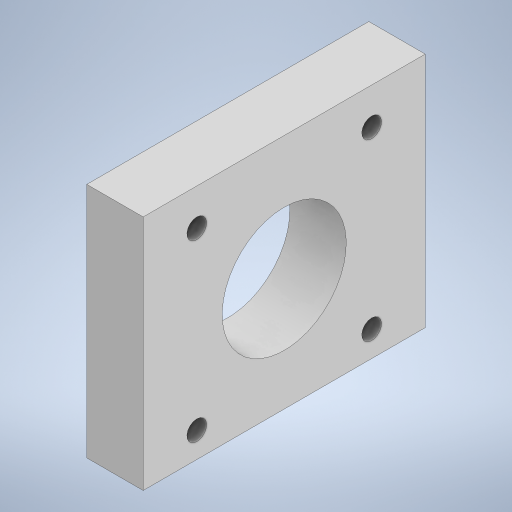
# Autodesk Inventor part: staffa motore
Saved by Autodesk Inventor 2024 (Build 280153000, 153)
## iProperties
Created: 2024-03-01
Part Number: staffa motore
Material: Generico
Document SubType Name: Modeling
Designer: Giorgio
Density: 1 g/cm^3
Appearance: Default
Author: Giorgio
Autodesk Inventor part; units mm, degrees
ref_plane "YZ Plane" through (0, 0, 0) normal (1, 0, 0) x (0, 1, 0)
ref_plane "XZ Plane" through (0, 0, 0) normal (0, 1, 0) x (-1, 0, 0)
ref_plane "XY Plane" through (0, 0, 0) normal (0, 0, 1) x (1, 0, 0)
sketch "Schizzo1" plane through (0, 0, 0) normal (1, 0, 0) x (0, 1, 0)
  circle A0 centre (57.5242, -67.0257) radius 11
  line L0 (37.5242, -92.0257) -> (79.5242, -92.0257)
  line L1 (79.5242, -92.0257) -> (79.5242, -42.0257)
  line L2 (79.5242, -42.0257) -> (37.5242, -42.0257)
  line L3 (37.5242, -42.0257) -> (37.5242, -92.0257)
  circle A1 centre (42.0242, -82.5257) radius 1.75
  circle A2 centre (42.0242, -51.5257) radius 1.75
  circle A3 centre (73.0242, -51.5257) radius 1.75
  circle A4 centre (73.0242, -82.5257) radius 1.75
  point P0 (0, 0)
  point P1 (79.5242, -67.0257)
  dimension "d0" = 22
  dimension "d1" = 42
  dimension "d2" = 50
  dimension "d4" = 31
  dimension "d5" = 31
  dimension "d6" = 15.5
  dimension "d7" = 31
  dimension "d8" = 31
  dimension "d9" = 0
  dimension "d10" = 15.5
  dimension "d11" = 0
  dimension "d12" = 3.5
  dimension "d13" = 3.5
  dimension "d14" = 3.5
  dimension "d15" = 3.5
  dimension "d16" = 22
  dimension "d17" = 25
  constraints: 8 end point, 5 centre point, 2 parallel, 1 horizontal, 1 midpoint, 1 perpendicular
  measures "d0" diameter of A0
  measures "d1" distance of L2.end L1.end
  measures "d2" distance of L1.end L0.end
  measures "d4" distance of A4.centre A1.centre
  measures "d5" distance of A3.centre A2.centre
  measures "d6" horizontal distance of A0.centre A2.centre
  measures "d7" distance of A1.centre A2.centre
  measures "d8" distance of A4.centre A3.centre
  measures "d9" horizontal distance of A2.centre A1.centre
  measures "d10" horizontal distance of A0.centre A4.centre
  measures "d11" vertical distance of A4.centre A1.centre
  measures "d12" diameter of A1
  measures "d13" diameter of A2
  measures "d14" diameter of A3
  measures "d15" diameter of A4
  measures "d16" distance of point (79.524, -67.026) A0.centre
  measures "d17" distance from line of L0 A0.centre
extrude "Estrusione1" add sketch "Schizzo1" along normal blind 10
equation "\"d5\" = d4"
equation "\"d6\" = 0.5 * d4"
equation "\"d7\" = d4"
equation "\"d8\" = d4"
equation "\"d10\" = 0.5 * d4"
equation "\"d13\" = d12"
equation "\"d14\" = d12"
equation "\"d15\" = d12"
equation "\"d17\" = 0.5 * d2"
